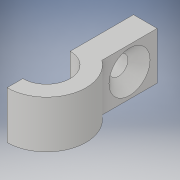
# Autodesk Inventor part: miniWiresHolder
Saved by Autodesk Inventor 2019 (Build 230136000, 136)
## iProperties
Created: 2019-08-24
Part Number: miniWiresHolder
Material: Generic
Document SubType Name: Modeling
Designer: fablab
Density: 1 g/cm^3
Appearance: Default
Author: fablab
Autodesk Inventor part; units mm, degrees
ref_plane "YZ Plane" through (0, 0, 0) normal (1, 0, 0) x (0, 1, 0)
ref_plane "XZ Plane" through (0, 0, 0) normal (0, 1, 0) x (-1, 0, 0)
ref_plane "XY Plane" through (0, 0, 0) normal (0, 0, 1) x (1, 0, 0)
sketch "Sketch1" plane through (0, 0, 0) normal (0, 1, 0) x (-1, 0, 0)
  arc A0 (0, 1.5) -> (0, -1.5) centre (0, 0) ccw
  line L0 (0, 1.5) -> (0, 2.5)
  arc A1 (0, 2.5) -> (0, -2.5) centre (0, 0) ccw
  line L1 (0, -1.5) -> (0, -2.5)
  line L2 (0, -2.5) -> (-1.5, -2.5)
  line L3 (-1.5, -2.5) -> (-1.5, -5.5)
  line L4 (-1.5, -5.5) -> (0, -5.5)
  line L5 (0, -5.5) -> (0, -2.5)
  line L6 (-1.5, -2.5) -> (-1.5, -2)
  dimension "d0" = 1.5
  dimension "d1" = 1
  dimension "d2" = 1.5
  dimension "d3" = 3
  constraints: 14 end point, 5 point on circle, 3 vertical, 2 centre point, 2 coincident, 2 parallel, 1 horizontal, 1 perpendicular
  measures "d0" radius of A0
  measures "d1" distance of L0.start L0.end
  measures "d2" distance of L4.end L3.end
  measures "d3" distance of L3.end L2.end
extrude "Extrusion1" add sketch "Sketch1" along normal blind 3
sketch "Sketch2" plane through (1.5, 0, -2) normal (1, 0, 0) x (0, 0, -1)
  line L0 (0, 3) -> (3.5, 3) projected
  line L1 (1.75, 3) -> (1.75, 0) construction
  line L2 (3.5, 0) -> (3.5, 3) projected
  line L3 (3.5, 1.5) -> (1.75, 1.5) construction
  circle A0 centre (1.75, 1.5) radius 0.6
  point P0 (-2, 0)
  dimension "d6" = 1.2
  constraints: 4 end point, 3 midpoint, 1 centre point, 1 coincident, 1 vertical
  measures "d6" diameter of A0
extrude "Extrusion2" cut sketch "Sketch2" against normal blind 3
chamfer "Chamfer1" distance 0.7 angle 45 1 edges at (1.5, 1.5, -3.15)
body "Solid1"
